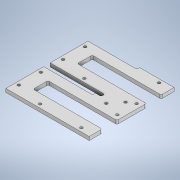
# Autodesk Inventor part: Battery Top Plate
Saved by Autodesk Inventor 2021 (Build 250183000, 183)
## iProperties
Created: 2020-08-13
Part Number: Battery Top Plate
Material: Generic
Document SubType Name: Modeling
Designer: jgray
Density: 1 g/cm^3
Appearance: Default
Author: jgray
Autodesk Inventor part; units mm, degrees
ref_plane "YZ Plane" through (0, 0, 0) normal (1, 0, 0) x (0, 1, 0)
ref_plane "XZ Plane" through (0, 0, 0) normal (0, 1, 0) x (-1, 0, 0)
ref_plane "XY Plane" through (0, 0, 0) normal (0, 0, 1) x (1, 0, 0)
sketch "Sketch1" plane through (0, 0, 0) normal (0, 1, 0) x (-1, 0, 0)
  line L0 (0, 0) -> (116.2, 0)
  line L1 (116.2, 0) -> (116.2, -56.7)
  line L2 (116.2, -56.7) -> (42, -56.7)
  line L3 (2, -18) -> (94.2, -18)
  line L4 (96.2, -20) -> (96.2, -36.75)
  line L5 (94.2, -38.75) -> (2, -38.75)
  arc A0 (96.2, -20) -> (94.2, -18) centre (94.2, -20) ccw
  arc A1 (94.2, -38.75) -> (96.2, -36.75) centre (94.2, -36.75) ccw
  line L6 (0, -56.75) -> (0, -40.75)
  line L7 (0, -16) -> (0, 0)
  arc A2 (0, -16) -> (2, -18) centre (2, -16) ccw
  arc A3 (2, -38.75) -> (0, -40.75) centre (2, -40.75) ccw
  line L8 (151.2965, -59.25) -> (-22.324, -59.25) construction
  line L9 (0, -118.5) -> (116.2, -118.5)
  line L10 (116.2, -118.5) -> (116.2, -61.8)
  line L11 (116.2, -61.8) -> (42, -61.8)
  line L12 (2, -100.5) -> (94.2, -100.5)
  line L13 (96.2, -98.5) -> (96.2, -81.75)
  line L14 (94.2, -79.75) -> (2, -79.75)
  arc A4 (94.2, -100.5) -> (96.2, -98.5) centre (94.2, -98.5) ccw
  arc A5 (96.2, -81.75) -> (94.2, -79.75) centre (94.2, -81.75) ccw
  line L15 (0, -61.75) -> (0, -77.75)
  line L16 (0, -102.5) -> (0, -118.5)
  arc A6 (2, -100.5) -> (0, -102.5) centre (2, -102.5) ccw
  arc A7 (0, -77.75) -> (2, -79.75) centre (2, -77.75) ccw
  line L17 (40, -58.7) -> (40, -59.8)
  line L18 (0, -61.75) -> (0, -56.75)
  arc A8 (40, -59.8) -> (42, -61.8) centre (42, -59.8) ccw
  arc A9 (42, -56.7) -> (40, -58.7) centre (42, -58.7) ccw
  point P0 (96.2, -38.75)
  point P1 (96.2, -18)
  point P2 (0, -38.75)
  point P3 (0, -28.375)
  point P4 (96.2, -79.75)
  point P5 (96.2, -100.5)
  point P6 (0, -79.75)
  point P7 (0, -90.125)
  dimension "d3" = 20.75
  dimension "d4" = 2
  dimension "d11" = 2
  dimension "d26" = 2
  dimension "d27" = 59.25
  dimension "d28" = 59.25
  dimension "d29" = 116.2
  dimension "d30" = 20
  dimension "d31" = 5.1
  dimension "d32" = 2.55
  dimension "d33" = 40
  dimension "d34" = 18
  constraints: 38 end point, 20 point on circle, 20 symmetric about line, 12 point on line, 12 tangent, 10 centre point, 5 parallel, 3 equal radius, 3 horizontal, 2 perpendicular, 1 collinear, 4 other
  measures "d3" distance of point (96.2, -18) point (96.2, -38.75)
  measures "d4" radius of A0
  measures "d11" radius of A2
  measures "d26" radius of A8
  measures "d27" distance between parallel lines of L0 L8
  measures "d28" distance between parallel lines of L9 L8
  measures "d29" distance between parallel lines of L16 L10
  measures "d30" distance between parallel lines of L10 L13
  measures "d31" distance between parallel lines of L11 L2
  measures "d32" distance between parallel lines of L2 L8
  measures "d33" distance between parallel lines of L16 L17
  measures "d34" distance between parallel lines of L9 L12
extrude "Extrusion1" add sketch "Sketch1" along normal blind 5
sketch "Sketch3" plane through (0, 5, 0) normal (0, 1, 0) x (1, 0, 0)
  line L0 (-141.9344, 59.25) -> (33.9299, 59.25) construction
  line L1 (0, 40.75) -> (0, 77.75) construction
  line L2 (-141.9344, 66.75) -> (21.3081, 66.75) construction
  line L3 (-111.2, -34.402) -> (-111.2, 125.7551) construction
  line L4 (-130.4345, 113.5) -> (5.6009, 113.5) construction
  line L5 (-141.9344, 5) -> (8.4057, 5) construction
  line L6 (-116.2, 0) -> (0, 0) construction
  line L7 (0, 118.5) -> (-116.2, 118.5) construction
  line L8 (-150.0685, 51.75) -> (12.052, 51.75) construction
  line L9 (-16, -62.5764) -> (-16, 180.6044) construction
  line L10 (0, 102.5) -> (0, 118.5) construction
  line L11 (-73.5, -39.5766) -> (-73.5, 137.6901) construction
  line L12 (-73.5, -38.2066) -> (-73.5, 155.6811) construction
  line L13 (-116.2, 56.7) -> (-116.2, 0) projected
  point P0 (0, 59.25)
  point P1 (-111.2, 13)
  point P2 (-111.2, 43.75)
  point P3 (-111.2, 74.75)
  point P4 (-111.2, 105.5)
  point P5 (-16, 5)
  point P6 (-16, 113.5)
  point P7 (-16, 66.75)
  point P8 (-73.5, 66.75)
  point P9 (-28, 51.75)
  point P10 (-73.5, 5)
  dimension "d35" = 5
  dimension "d36" = 5
  dimension "d37" = 7.5
  dimension "d38" = 13
  dimension "d39" = 15.5
  dimension "d40" = 15.5
  dimension "d41" = 13
  dimension "d42" = 7.5
  dimension "d43" = 16
  dimension "d44" = 12
  dimension "d45" = 73.5
  dimension "d53" = 73.5
  dimension "d54" = 5
  constraints: 18 end point, 16 point on line, 4 vertical, 3 parallel, 2 horizontal, 1 midpoint
  measures "d35" distance between parallel lines of L5 L6
  measures "d36" distance between parallel lines of L7 L4
  measures "d37" distance between parallel lines of L0 L2
  measures "d38" distance from line of point (-111.2, 105.5) L7
  measures "d39" distance from line of point (-111.2, 74.75) L0
  measures "d40" distance from line of point (-111.2, 43.75) L0
  measures "d41" distance from line of point (-111.2, 13) L6
  measures "d42" distance between parallel lines of L8 L0
  measures "d43" distance between parallel lines of L9 L10
  measures "d44" distance from line of point (-28, 51.75) L9
  measures "d45" distance between parallel lines of L10 L11
  measures "d53" distance between parallel lines of L10 L12
  measures "d54" distance between parallel lines of L13 L3
hole "Hole1" at (-111.2, 5, -13) at (-111.2, 5, -43.75) at (-111.2, 5, -74.75) at (-111.2, 5, -105.5) at (-16, 5, -5) at (-16, 5, -113.5) at (-16, 5, -66.75) at (-73.5, 5, -66.75) at (-28, 5, -51.75) at (-73.5, 5, -5) direction (0, -1, 0) diameter 3.8 end through all
sketch "Sketch4" plane through (0, 5, 0) normal (0, 1, 0) x (1, 0, 0)
  line L0 (-116.2, 52.75) -> (-49, 52.75)
  line L1 (-48, 53.75) -> (-48, 64.75)
  line L2 (-49, 65.75) -> (-116.2, 65.75)
  line L3 (-116.2, 65.75) -> (-116.2, 52.75)
  line L4 (-144.8708, 59.25) -> (29.3106, 59.25) construction
  line L5 (-40, 59.8) -> (-40, 58.7) construction
  line L6 (0, 40.75) -> (0, 77.75) projected
  line L7 (0, 102.5) -> (0, 118.5) projected
  arc A0 (-48, 64.75) -> (-49, 65.75) centre (-49, 64.75) ccw
  arc A1 (-49, 52.75) -> (-48, 53.75) centre (-49, 53.75) ccw
  line L8 (-116.2, 59.25) -> (-48, 59.25)
  line L9 (0, 118.5) -> (-116.2, 118.5) projected
  line L10 (-116.2, 118.5) -> (-48, 118.5)
  line L11 (-48, 118.5) -> (-48, 115.5)
  line L12 (-49, 114.5) -> (-116.2, 114.5)
  line L13 (-116.2, 114.5) -> (-116.2, 118.5)
  arc A2 (-49, 114.5) -> (-48, 115.5) centre (-49, 115.5) ccw
  circle A3 centre (-28, 51.75) radius 1.9 projected
  circle A4 centre (-16, 66.75) radius 1.9 projected
  circle A5 centre (-16, 5) radius 1.9 projected
  circle A6 centre (-111.2, 74.75) radius 1.9 projected
  circle A7 centre (-111.2, 13) radius 1.9 projected
  circle A8 centre (-111.2, 43.75) radius 1.9 projected
  circle A9 centre (-111.2, 105.5) radius 1.9 projected
  circle A10 centre (-16, 113.5) radius 1.9 projected
  circle A11 centre (-73.5, 66.75) radius 1.9 projected
  circle A12 centre (-73.5, 5) radius 1.9 projected
  line L14 (-2, 18) -> (-94.2, 18) projected
  arc A13 (-96.2, 20) -> (-94.2, 18) centre (-94.2, 20) ccw projected
  line L15 (-96.2, 20) -> (-96.2, 36.75) projected
  arc A14 (-94.2, 38.75) -> (-96.2, 36.75) centre (-94.2, 36.75) ccw projected
  line L16 (-94.2, 38.75) -> (-2, 38.75) projected
  arc A15 (-2, 38.75) -> (0, 40.75) centre (-2, 40.75) ccw projected
  line L17 (0, 40.75) -> (0, 77.75) projected
  arc A16 (0, 77.75) -> (-2, 79.75) centre (-2, 77.75) ccw projected
  line L18 (-2, 79.75) -> (-94.2, 79.75) projected
  arc A17 (-96.2, 81.75) -> (-94.2, 79.75) centre (-94.2, 81.75) ccw projected
  line L19 (-96.2, 81.75) -> (-96.2, 98.5) projected
  arc A18 (-94.2, 100.5) -> (-96.2, 98.5) centre (-94.2, 98.5) ccw projected
  line L20 (-94.2, 100.5) -> (-2, 100.5) projected
  arc A19 (-2, 100.5) -> (0, 102.5) centre (-2, 102.5) ccw projected
  line L21 (0, 102.5) -> (0, 118.5) projected
  line L22 (0, 118.5) -> (-116.2, 118.5) projected
  line L23 (-116.2, 118.5) -> (-116.2, 61.8) projected
  line L24 (-116.2, 61.8) -> (-42, 61.8) projected
  arc A20 (-40, 59.8) -> (-42, 61.8) centre (-42, 59.8) ccw projected
  line L25 (-40, 59.8) -> (-40, 58.7) projected
  arc A21 (-42, 56.7) -> (-40, 58.7) centre (-42, 58.7) ccw projected
  line L26 (-42, 56.7) -> (-116.2, 56.7) projected
  line L27 (-116.2, 56.7) -> (-116.2, 0) projected
  line L28 (-116.2, 0) -> (0, 0) projected
  line L29 (0, 0) -> (0, 16) projected
  arc A22 (0, 16) -> (-2, 18) centre (-2, 16) ccw projected
  point P0 (-40, 59.25)
  dimension "d55" = 48
  dimension "d57" = 6.5
  dimension "d58" = 13
  dimension "d64" = 4
  constraints: 20 end point, 7 point on line, 6 point on circle, 6 tangent, 4 parallel, 3 centre point, 3 collinear, 3 horizontal, 3 midpoint, 2 perpendicular
  measures "d55" distance between parallel lines of L6 L1
  measures "d57" distance between parallel lines of L2 L4
  measures "d58" distance between parallel lines of L2 L0
  measures "d64" distance between parallel lines of L10 L12
extrude "Extrusion2" cut sketch "Sketch4" against normal blind 5 contours L3 L26 L1 A1 L0 | L3 L8 L1 L26 | L13 L9 L11 A2 L12
sketch "Sketch5" plane through (0, 5, 0) normal (0, 1, 0) x (1, 0, 0)
  line L0 (-6.5, 90.3299) -> (-6.5, 26.5621) construction
  line L1 (0, 40.75) -> (0, 77.75) projected
  line L2 (-18, 59.25) -> (18, 59.25) construction
  point P0 (0, 0)
  point P1 (0, 59.25)
  point P2 (0, 59.25)
  point P3 (-6.5, 72.75)
  point P4 (-6.5, 45.75)
  dimension "d66" = 6.5
  dimension "d67" = 13.5
  dimension "d68" = 13.5
  constraints: 4 end point, 4 midpoint, 2 point on line, 1 horizontal, 1 vertical
  measures "d66" distance between parallel lines of L0 L1
  measures "d67" distance from line of point (-6.5, 72.75) L2
  measures "d68" distance from line of point (-6.5, 45.75) L2
hole "Hole2" at (-6.5, 5, -72.75) at (-6.5, 5, -45.75) direction (0, -1, 0) diameter 3.8 end through all
body "Solid1"
